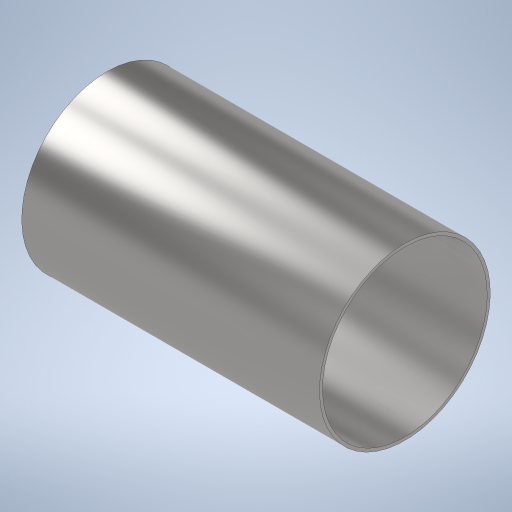
# Autodesk Inventor part: stainless steel final chamber
Saved by Autodesk Inventor 2023 (Build 270158000, 158)
## iProperties
Created: 2022-09-19
Part Number: stainless steel final chamber
Material: Stainless Steel
Document SubType Name: Modeling
Designer: station
Density: 8 g/cm^3
Appearance: Semi-Polished
Author: station
Autodesk Inventor part; units mm, degrees
ref_plane "YZ Plane" through (0, 0, 0) normal (1, 0, 0) x (0, 1, 0)
ref_plane "XZ Plane" through (0, 0, 0) normal (0, 1, 0) x (-1, 0, 0)
ref_plane "XY Plane" through (0, 0, 0) normal (0, 0, 1) x (1, 0, 0)
sketch "Sketch1" plane through (0, 0, 0) normal (0, 0, 1) x (1, 0, 0)
  line L0 (0, 0) -> (200, 0) construction
  line L1 (0, 0) -> (0, 54.5) construction
  line L2 (0, 54.5) -> (192, 54.5)
  line L3 (192, 54.5) -> (192, 0) construction
  line L4 (196, 0) -> (196, 56.5) construction
  line L5 (192, 56.5) -> (-2, 56.5)
  line L6 (-2, 56.5) -> (-2, -2) construction
  line L7 (-2, -2) -> (200, -2) construction
  line L8 (192, 54.5) -> (192, 56.5)
  line L9 (0, 54.5) -> (-5, 54.5)
  line L10 (-5, 54.5) -> (-5, 56.5)
  line L11 (-5, 56.5) -> (-2, 56.5)
  dimension "d7" = 54.5
  dimension "d8" = 192
  dimension "d9" = 200
  dimension "d10" = 2
  dimension "d11" = 5
  constraints: 24 end point, 6 perpendicular, 3 vertical, 1 horizontal, 1 point on line, 1 other
  measures "d7" distance of L0.start L1.end
  measures "d8" distance of L1.end L2.end
  measures "d9" distance of L0.start L0.end
  measures "d10" distance between parallel lines of L2 L5
  measures "d11" distance of L1.end L9.end
revolve "Revolution1" add sketch "Sketch1" angle 360 about axis through (0, 0, 0) along (1, 0, 0)
body "Solid1"
